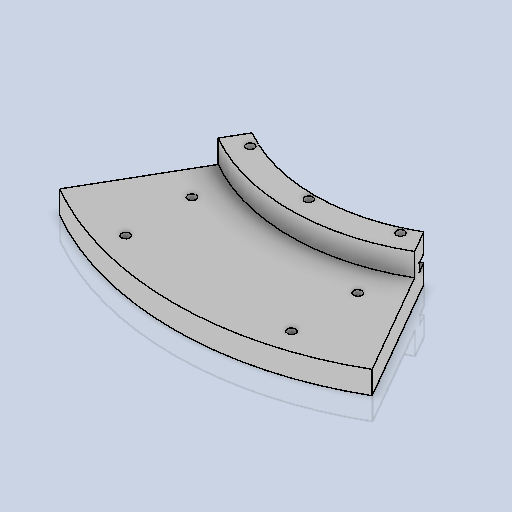
# Autodesk Inventor part: shelf_attachment
Saved by Autodesk Inventor 2026.1 (Build 301233000, 233)
## iProperties
Created: 2025-08-31
Part Number: shelf_attachment
Material: Generic
Document SubType Name: Modeling
Designer: baseb
Density: 1 g/cm^3
Appearance: Default
Author: baseb
Autodesk Inventor part; units mm, degrees
ref_plane "YZ Plane" through (0, 0, 0) normal (1, 0, 0) x (0, 1, 0)
ref_plane "XZ Plane" through (0, 0, 0) normal (0, 1, 0) x (-1, 0, 0)
ref_plane "XY Plane" through (0, 0, 0) normal (0, 0, 1) x (1, 0, 0)
sketch "Sketch1" plane through (0, 0, 0) normal (1, 0, 0) x (0, 1, 0)
  line L0 (-17.4625, 9.525) -> (17.4625, 9.525)
  line L1 (17.4625, 9.525) -> (17.4625, -9.525)
  line L2 (17.4625, -9.525) -> (-17.4625, -9.525)
  line L3 (-17.4625, -9.525) -> (-17.4625, 9.525)
  line L4 (-17.4625, 9.525) -> (17.4625, -9.525) construction
  line L5 (17.4625, 9.525) -> (-17.4625, -9.525) construction
  line L6 (3.175, -9.525) -> (3.175, 0)
  line L7 (3.175, 0) -> (-3.175, 0)
  line L8 (-3.175, 0) -> (-3.175, -9.525)
  line L9 (-17.4625, 9.525) -> (0, 9.525)
  line L10 (0, 9.525) -> (0, 98.425)
  line L11 (0, 98.425) -> (-17.4625, 98.425)
  line L12 (-17.4625, 98.425) -> (-17.4625, 9.525)
  line L13 (0, -9.525) -> (-0.0003, -140.97) construction
  line L14 (-0.0003, -140.97) -> (69.3079, -140.97)
  point P0 (0, 0)
  point P1 (0, 0)
  dimension "d0" = 6.35
  dimension "d1" = 9.525
  dimension "d2" = 9.525
  dimension "d3" = 19.05
  dimension "d4" = 34.925
  dimension "d5" = 0
  dimension "d6" = 88.9
  dimension "d7" = 131.445
  constraints: 30 end point, 5 parallel, 4 midpoint, 3 horizontal, 2 perpendicular, 2 point on line
  measures "d0" distance of L6.end L7.end
  measures "d1" distance of L6.start L6.end
  measures "d2" distance of L7.end L8.end
  measures "d3" distance of L0.end L1.end
  measures "d4" distance of L0.start L0.end
  measures "d5" distance of point (0, 0) point (0, 0)
  measures "d6" distance of L9.end L10.end
  measures "d7" distance of L13.start L13.end
revolve "Revolution1" add sketch "Sketch1" angle 60 mid plane about axis through (0, -0.0003, -140.97) along (0, 1, 0) contours L12 L11 L10 L0 | L0 L1 L2 L6 L7 L8 L3
sketch "Sketch2" plane through (-75.2475, 17.4625, -10.6375) normal (0, 1, 0) x (0.8660254, 0, 0.5)
  arc A0 (70.485, 28.4114) -> (122.0836, 80.01) centre (0, 150.495) ccw projected
  arc A1 (0, 19.05) -> (113.8347, 84.7725) centre (0, 150.495) ccw projected
  line L0 (0, 19.05) -> (0, 0) construction
  line L1 (113.8347, 84.7725) -> (122.0836, 80.01) construction
  arc A2 (89.2238, 47.5795) -> (117.9592, 82.3912) centre (0, 150.495) ccw construction
  circle A3 centre (11.8618, 14.805) radius 3.175
  circle A4 centre (68.0955, 32.5311) radius 3.175
  circle A5 centre (111.5692, 72.3618) radius 3.175
  point P0 (0, 0)
  dimension "d22" = 140.97
  dimension "d23" = 136.2075
  dimension "d24" = 6.35
  dimension "d25" = 11.8618
  dimension "d34" = 50
  constraints: 4 centre point, 3 point on circle, 1 midpoint, 6 other
  measures "d22" radius of A0
  measures "d23" radius of A2
  measures "d24" diameter of A3
extrude "Extrusion2" cut sketch "Sketch2" against normal up to surface (14.2875 mm away)
sketch "Sketch3" plane through (0, 0, -140.97) normal (0, 1, 0) x (1, 0, 0)
  line L0 (-63.5, -212.9652) -> (63.5, -212.9652) construction
  line L1 (63.5, -212.9652) -> (63.5, -162.1652) construction
  line L2 (63.5, -162.1652) -> (-63.5, -162.1652) construction
  line L3 (-63.5, -162.1652) -> (-63.5, -212.9652) construction
  line L4 (-63.5, -212.9652) -> (63.5, -162.1652) construction
  line L5 (63.5, -212.9652) -> (-63.5, -162.1652) construction
  line L6 (-75.2475, -130.3325) -> (-119.6975, -207.3222) projected
  line L7 (75.2475, -130.3325) -> (119.6975, -207.3222) projected
  arc A0 (-97.4725, -168.8273) -> (97.4725, -168.8273) centre (0, 75.3248) ccw construction
  circle A1 centre (63.5, -162.1652) radius 3.175
  circle A2 centre (-63.5, -162.1652) radius 3.175
  circle A3 centre (63.5, -212.9652) radius 3.175
  circle A4 centre (-63.5, -212.9652) radius 3.175
  point P0 (0, -140.97)
  point P1 (0, -187.5652)
  dimension "d37" = 50.8
  dimension "d38" = 127
  dimension "d39" = 262.89
  dimension "d41" = 6.35
  dimension "d44" = 127
  dimension "d47" = 50.8
  constraints: 12 end point, 5 centre point, 4 midpoint, 2 horizontal, 2 parallel, 2 point on circle, 1 coincident, 1 perpendicular, 1 vertical, 6 other
  measures "d37" distance of L2.end L0.start
  measures "d38" distance of L1.end L2.end
  measures "d39" radius of A0
  measures "d41" diameter of A1
  measures "d44" distance of A1.centre A2.centre
  measures "d47" distance of A1.centre A3.centre
extrude "Extrusion3" cut sketch "Sketch3" against normal through all
equation "\"d2\" = d1"
equation "\"d3\" = 2 * d1"
body "Solid1"
